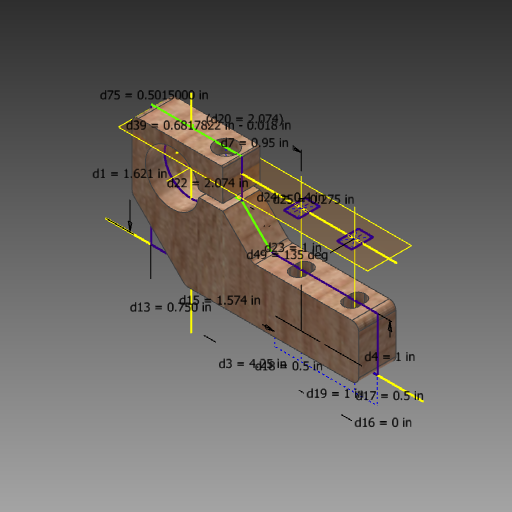
# Autodesk Inventor part: J005363
Saved by Autodesk Inventor 2018.2 (Build 222227000, 227)
## iProperties
Created: 2015-08-05
Material: ALUMINUM, 6061-T651
Vendor: HHMI: JRC - ID&F
Document SubType Name: Modeling
Designer: ARNOLDJ
Density: 2.7 g/cm^3
Appearance: Birch - Natural Polished
Part Number: J005363
Description: MBS OUTER EM MOUNT
Project: P-201804
RuleStatus: InUse
AfterDocSave0: file://Part Number Cleaner
LAB/DEPT: SVOBODA (LAB)
REQUESTING SCIENTIST: SOFRONIEW, NICK
SURFACE ROUGHNESS: 63 Ra
DESIGN DEPARTMENT: HHMI: JRC - ID&F
SPECIAL FINISH: ANODIZE PER MIL-A-8625F, TYPE II, CLASS 2 (BLACK)
ALTERED ITEM PART NUMBER: N/A
ALTERED ITEM VENDOR: N/A
ALTERED ITEM DESCRIPTION: N/A
Revision Number: -
Autodesk Inventor part; units mm, degrees
note: some values were not read from the file. Chosen so that the rebuilt part matches the saved one: direction of "Hole2".
ref_plane "YZ Plane" through (0, 0, 0) normal (1, 0, 0) x (0, 1, 0)
sketch "Sketch1" plane through (0, 0, 0) normal (0, 0, 1) x (1, 0, 0)
  line L0 (0, 71.9938) -> (0, -26.8156) projected
  line L1 (-40.64, 0) -> (110.49, 0) projected
  line L2 (-19.05, 0) -> (-19.05, 57.8782)
  line L3 (24.13, 57.8782) -> (24.13, 39.5859)
  line L4 (-19.05, 0) -> (88.9, 0)
  line L5 (88.9, 0) -> (88.9, 25.4)
  line L6 (0, 41.1734) -> (24.13, 41.1734) construction
  line L7 (12.6388, 39.5859) -> (24.13, 39.5859)
  line L8 (24.13, 39.5859) -> (24.13, 42.7577)
  line L9 (24.13, 42.7577) -> (12.6392, 42.7577)
  line L10 (4.9628, 39.5889) -> (24.13, 42.7577) construction
  line L11 (24.13, 39.5859) -> (4.9638, 42.7609) construction
  line L12 (39.9796, 0) -> (88.9, 0) construction
  line L13 (88.9, 0) -> (88.9, -12.7) construction
  line L14 (88.9, -12.7) -> (39.9796, -12.7) construction
  line L15 (39.9796, -12.7) -> (39.9796, 0) construction
  line L16 (52.6796, -12.7) -> (52.6796, 0) construction
  line L17 (78.0796, -12.7) -> (78.0796, 0) construction
  line L18 (38.3159, 25.4) -> (88.9, 25.4)
  line L19 (16.8601, 41.1734) -> (16.8601, 57.8782) construction
  line L20 (12.7635, 41.1734) -> (12.7635, 34.371) construction
  line L21 (24.13, 39.5859) -> (38.3159, 25.4)
  line L22 (-19.05, 57.8782) -> (24.13, 57.8782)
  arc A0 (12.6392, 42.7577) -> (12.6388, 39.5859) centre (0, 41.1734) ccw
  point P0 (14.5469, 41.1734)
  dimension "d1" = 41.1734
  dimension "d3" = 107.95
  dimension "d4" = 25.4
  dimension "d7" = 24.13
  dimension "d13" = 19.05
  dimension "d15" = 39.9796
  dimension "d16" = 0
  dimension "d17" = 12.7
  dimension "d18" = 12.7
  dimension "d19" = 25.4
  dimension "d20" = 52.6796
  dimension "d39" = 16.8601
  dimension "d49" = 135
  dimension "d75" = 12.7381
  constraints: 42 end point, 14 point on line, 7 perpendicular, 3 horizontal, 3 parallel, 2 point on circle, 2 vertical, 1 centre point, 1 coincident, 1 midpoint
  measures "d1" distance from line of L1 L6.start
  measures "d3" distance of L2.start L4.end
  measures "d4" distance of L4.end L5.end
  measures "d7" distance between parallel lines of L3 L0
  measures "d13" distance between parallel lines of L0 L2
  measures "d15" distance between parallel lines of L15 L0
  measures "d16" distance between parallel lines of L13 L5
  measures "d17" distance of L14.end L12.start
  measures "d18" distance between parallel lines of L16 L15
  measures "d19" distance between parallel lines of L17 L16
  measures "d20" distance between parallel lines of L16 L0
  measures "d39" distance between parallel lines of L0 L19
  measures "d49" angle of L18 L21
  measures "d75" radius of A0
extrude "Extrusion1" add sketch "Sketch1" along normal mid plane 17.78 contours L22 L3 L9 A0 L0 | L0 A0 L1 L2 L22 | A0 L7 L21 L18 L5 L1 L0
ref_plane "Work Plane1" through (0, 50.8, 0) normal (0, 1, 0) x (-1, 0, 0)
sketch "Sketch2" plane through (0, 50.8, 0) normal (0, 1, 0) x (-1, 0, 0)
  line L0 (0, -7.112) -> (0, 7.112) projected
  line L1 (-97.8865, 0) -> (16.3144, 0) projected
  line L2 (-56.1721, 5.08) -> (-49.1871, 5.08)
  line L3 (-49.1871, 5.08) -> (-49.1871, -5.08)
  line L4 (-49.1871, -5.08) -> (-56.1721, -5.08)
  line L5 (-56.1721, -5.08) -> (-56.1721, 5.08)
  line L6 (-56.1721, 5.08) -> (-49.1871, -5.08) construction
  line L7 (-49.1871, 5.08) -> (-56.1721, -5.08) construction
  line L8 (-81.5721, 5.08) -> (-74.5871, 5.08)
  line L9 (-74.5871, 5.08) -> (-74.5871, -5.08)
  line L10 (-74.5871, -5.08) -> (-81.5721, -5.08)
  line L11 (-81.5721, -5.08) -> (-81.5721, 5.08)
  line L12 (-81.5721, 5.08) -> (-74.5871, -5.08) construction
  line L13 (-74.5871, 5.08) -> (-81.5721, -5.08) construction
  point P0 (0, 0)
  point P1 (-52.6796, 0)
  point P2 (-78.0796, 0)
  dimension "d22" = 52.6796
  dimension "d23" = 25.4
  dimension "d24" = 10.16
  dimension "d25" = 6.985
  constraints: 24 end point, 4 midpoint, 4 parallel, 3 point on line, 2 horizontal, 2 perpendicular, 1 collinear
  measures "d22" distance from line of point (-52.68, 0) L0
  measures "d23" distance of point (-78.08, 0) point (-52.68, 0)
  measures "d24" distance of L2.end L3.end
  measures "d25" distance of L3.end L4.end
extrude "Extrusion2" cut sketch "Sketch2" against normal up to next
sketch "Sketch3" plane through (0, 0, 0) normal (0, 0, 1) x (1, 0, 0)
  point P0 (0, 0)
fillet "Fillet1" radius 3.175 8 edges at (49.1871, 12.7, -5.08) (56.1721, 12.7, -5.08) (56.1721, 12.7, 5.08) (49.1871, 12.7, 5.08) (74.5871, 12.7, 5.08) (74.5871, 12.7, -5.08) (81.5721, 12.7, -5.08) (81.5721, 12.7, 5.08)
sketch "Sketch4" plane through (-19.05, 57.8782, 8.89) normal (0, 1, 0) x (1, 0, 0)
  line L0 (129.5216, 7.8564) -> (-21.59, 9.525)
  line L1 (43.18, 19.05) -> (43.18, 0)
  line L2 (19.05, 22.86) -> (19.05, -3.81)
  line L3 (116.9365, 8.89) -> (2.7356, 8.89) projected
  point P0 (19.05, 9.525)
  point P1 (129.5216, 7.8564)
  point P2 (-21.59, 9.525)
  point P3 (35.9156, 8.89)
  dimension "d38" = 16.8656
  dimension "d79" = 0
  constraints: 4 end point, 4 other
  measures "d38" distance from line of L2 point (35.916, 8.89)
  measures "d79" distance from line of L3 point (35.916, 8.89)
sketch "Sketch5" plane through (-19.05, 57.8782, 8.89) normal (0, 1, 0) x (1, 0, 0)
  point P0 (19.05, 9.525)
hole "Hole2" at (16.8656, 57.8782, 0) direction (0, -1, 0) diameter 5.4102 end up to surface counterbore diameter 10.541 counterbore depth 6.35
chamfer "Chamfer1" distance 25.4 angle 45 1 edges at (-19.05, 0, 0)
sketch "Sketch6" plane through (0, 0, 0) normal (1, 0, 0) x (0, 1, 0)
  line L0 (41.1734, -12.446) -> (41.1734, 12.446) projected
  line L1 (-11.5756, 0) -> (69.4538, 0) projected
  line L2 (28.4353, -4.7625) -> (28.1813, -4.7625)
  line L3 (28.1813, -4.7625) -> (28.1813, 4.7625)
  line L4 (28.1813, 4.7625) -> (28.4353, 4.7625)
  line L5 (28.4353, 4.7625) -> (28.4353, -4.7625)
  line L6 (28.4353, -4.7625) -> (28.1813, 4.7625) construction
  line L7 (28.1813, -4.7625) -> (28.4353, 4.7625) construction
  line L8 (28.4353, 8.89) -> (28.4353, -8.89) projected
  line L9 (57.8782, -8.89) -> (42.7577, -8.89) projected
  line L10 (42.7577, 8.89) -> (57.8782, 8.89) projected
  point P0 (0, 0)
  point P1 (28.3083, 0)
  dimension "d53" = 0
  dimension "d54" = 9.525
  dimension "d55" = 0.254
  dimension "d56" = 17.78
  constraints: 12 end point, 2 midpoint, 2 parallel, 1 horizontal, 1 perpendicular, 1 point on line
  measures "d53" distance between parallel lines of L8 L5
  measures "d54" distance of L4.end L2.start
  measures "d55" distance of L3.end L4.end
  measures "d56" distance between parallel lines of L9 L10
revolve "Revolution1" [suppressed]
hole "Hole3" at (16.8656, 39.5859, 0) direction (0, -1, 0) diameter 4.1402 depth 14.1986 tip angle 118
fillet "Fillet2" radius 0.254 2 edges at (12.6392, 42.7577, 0) (12.6388, 39.5859, 0)
fillet "Fillet3" radius 0.635 1 edges at (24.13, 57.8782, 0)
fillet "Fillet4" radius 3.175 5 edges at (-19.05, 57.8782, 0) (-19.05, 25.4, 0) (6.35, 0, 0) (88.9, 25.4, 0) (88.9, 0, 0)
chamfer "Chamfer2" [suppressed]
fillet "Fillet5" radius 3.175 1 edges at (38.3159, 25.4, 0)
body "Solid1"
